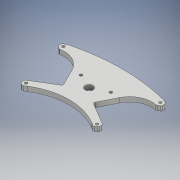
# Autodesk Inventor part: ステッピング固定具
Saved by Autodesk Inventor 2018 (Build 220112000, 112)
## iProperties
Created: 2018-08-16
Part Number: ステッピング固定具
Material: 一般
Document SubType Name: Modeling
Designer: shun2
Density: 1 g/cm^3
Appearance: 既定
Author: shun2
Autodesk Inventor part; units mm, degrees
ref_plane "YZ Plane" through (0, 0, 0) normal (1, 0, 0) x (0, 1, 0)
ref_plane "XZ Plane" through (0, 0, 0) normal (0, 1, 0) x (-1, 0, 0)
ref_plane "XY Plane" through (0, 0, 0) normal (0, 0, 1) x (1, 0, 0)
sketch "スケッチ1" plane through (0, 0, 0) normal (0, 0, 1) x (1, 0, 0)
  circle A0 centre (24.2131, 26.9091) radius 1.6
  circle A1 centre (8.9167, 85.9091) radius 1.6
  circle A2 centre (122.9167, 85.9091) radius 1.6
  circle A3 centre (107.6203, 26.9091) radius 1.6
  line L0 (65.9168, 92.271) -> (65.9166, 46.271)
  line L1 (107.6203, 25.1991) -> (107.6203, 28.6191)
  line L2 (22.5031, 26.9091) -> (25.9231, 26.9091)
  line L3 (24.2131, 25.1991) -> (24.2131, 28.6191)
  line L4 (7.2067, 85.9091) -> (10.6267, 85.9091)
  line L5 (8.9167, 84.1991) -> (8.9167, 87.6191)
  line L6 (124.6267, 85.9091) -> (121.2067, 85.9091)
  line L7 (122.9167, 84.1991) -> (122.9167, 87.6191)
  line L8 (109.3303, 26.9091) -> (105.9103, 26.9091)
  arc A4 (103.2949, 25.1358) -> (28.1968, 24.6091) centre (66.1769, -36.5761) ccw
  line L9 (6.0567, 82.7816) -> (8.3869, 81.4363)
  line L10 (5.0567, 86.8043) -> (5.0567, 84.5137)
  line L11 (123.7023, 81.4412) -> (126.0241, 82.7816)
  line L12 (110.2633, 24.5579) -> (108.2796, 23.4126)
  line L13 (103.2949, 25.1358) -> (106.2796, 23.4126)
  line L14 (28.1968, 24.6091) -> (25.2131, 22.8864)
  circle A5 centre (65.9167, 59.1833) radius 4.65
  circle A6 centre (65.9167, 67.1833) radius 14
  line L15 (82.734, 67.2168) -> (82.7592, 67.2168)
  circle A7 centre (48.4167, 67.2168) radius 1.6
  circle A8 centre (83.4167, 67.2168) radius 1.6
  arc A9 (37.9167, 67.2167) -> (9.7534, 81.2022) centre (14.5444, 55.5004) ccw
  arc A10 (122.3194, 81.2102) -> (93.9167, 67.2168) centre (117.3134, 55.5494) ccw
  line L16 (37.9167, 67.2167) -> (47.5918, 47.9164)
  line L17 (93.9167, 67.2168) -> (84.2485, 47.9303)
  arc A11 (46.8453, 45.3126) -> (47.5918, 47.9164) centre (45.8039, 47.0201) ccw
  arc A12 (84.2485, 47.9303) -> (85.0094, 45.3179) centre (86.0364, 47.034) ccw
  circle A13 centre (24.2131, 26.9091) radius 1.6
  circle A14 centre (107.6203, 26.9091) radius 1.6
  circle A15 centre (122.9167, 85.9091) radius 1.6
  circle A16 centre (8.9167, 85.9091) radius 1.6
  arc A17 (122.7823, 90.3275) -> (9.2985, 90.3275) centre (66.0404, -124.0864) ccw
  arc A18 (106.2796, 23.4126) -> (108.2796, 23.4126) centre (107.2796, 25.1447) ccw
  arc A19 (21.2294, 29.7864) -> (20.2294, 28.0543) centre (22.2294, 28.0543) ccw
  arc A20 (23.2131, 22.8864) -> (25.2131, 22.8864) centre (24.2131, 24.6185) ccw
  arc A21 (110.2633, 24.5579) -> (111.2633, 26.29) centre (109.2633, 26.29) ccw
  arc A22 (123.2706, 90.1261) -> (122.7823, 90.3275) centre (122.2706, 88.394) ccw
  arc A23 (126.0241, 82.7816) -> (127.0241, 84.5137) centre (125.0241, 84.5137) ccw
  arc A24 (122.3194, 81.2102) -> (123.7023, 81.4412) centre (122.7023, 83.1732) ccw
  arc A25 (9.2985, 90.3275) -> (8.8102, 90.1261) centre (9.8102, 88.394) ccw
  arc A26 (8.3869, 81.4363) -> (9.7534, 81.2022) centre (9.3869, 83.1683) ccw
  arc A27 (6.0567, 88.5363) -> (5.0567, 86.8043) centre (7.0567, 86.8043) ccw
  arc A28 (5.0567, 84.5137) -> (6.0567, 82.7816) centre (7.0567, 84.5137) ccw
  arc A29 (20.2294, 25.7638) -> (21.2294, 24.0317) centre (22.2294, 25.7638) ccw
  line L18 (8.8102, 90.1261) -> (6.0567, 88.5363)
  line L19 (123.2706, 90.1261) -> (126.0241, 88.5363)
  line L20 (20.2294, 28.0543) -> (20.2294, 25.7638)
  line L21 (21.2294, 24.0317) -> (23.2131, 22.8864)
  line L22 (46.8453, 45.3126) -> (21.2294, 29.7864)
  line L23 (85.0094, 45.3179) -> (110.2633, 30.3014)
  line L24 (111.2633, 26.29) -> (111.2633, 28.5694)
  line L25 (127.0241, 84.5137) -> (127.0241, 86.8043)
  arc A30 (127.0241, 86.8043) -> (126.0241, 88.5363) centre (125.0241, 86.8043) ccw
  arc A31 (111.2633, 28.5694) -> (110.2633, 30.3014) centre (109.2633, 28.5694) ccw
  point P0 (0, 0)
  dimension "d10" = 28
  dimension "d13" = 17.5
  dimension "d15" = 17.5
  dimension "d18" = 3.2
  dimension "d20" = 3.2
  dimension "d26" = 2
  dimension "d27" = 2.681
  dimension "d28" = 2.2906
  dimension "d29" = 2
  dimension "d31" = 2.2906
  dimension "d32" = 2
  constraints: 52 end point, 40 point on circle, 32 centre point, 15 tangent, 9 equal radius, 4 coincident, 3 vertical, 2 parallel, 1 horizontal, 1 point on line
  measures "d10" distance of L17.start A6.centre
  measures "d13" distance of A7.centre A6.centre
  measures "d15" distance of A8.centre A6.centre
  measures "d18" diameter of A14
  measures "d20" diameter of A16
  measures "d26" radius of A29
  measures "d27" distance of L11.start L11.end
  measures "d28" distance of L25.start L25.end
  measures "d29" radius of A24
  measures "d31" distance of L10.start L10.end
  measures "d32" radius of A31
extrude "押し出し1" add sketch "スケッチ1" along normal blind 5.5 contours A6 L0 A5 | L0 A5 A6 | A4 L14 A20 L21 A29 L20 A19 L22 A11 L16 A9 A26 L9 A28 L10 A27 L18 A25 A17 A22 L19 A30 L25 A23 L11 A24 A10 L17 A12 L23 A31 L24 A21 L12 A18 L13
